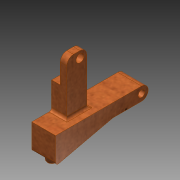
# Autodesk Inventor part: Swinging_connection
Saved by Autodesk Inventor 2015 (Build 190159000, 159)
## iProperties
Created: 2017-02-21
Part Number: Swinging_connection
Material: Wood (Cherry)
Document SubType Name: Modeling
Designer: Guy
Density: 0.63 g/cm^3
Appearance: Cherry - Natural Low Gloss
Author: Guy
Autodesk Inventor part; units mm, degrees
ref_plane "YZ Plane" through (0, 0, 0) normal (1, 0, 0) x (0, 1, 0)
ref_plane "XZ Plane" through (0, 0, 0) normal (0, 1, 0) x (-1, 0, 0)
ref_plane "XY Plane" through (0, 0, 0) normal (0, 0, 1) x (1, 0, 0)
sketch "Sketch1" plane through (0, 0, 0) normal (0, 0, 1) x (1, 0, 0)
  line L0 (0, 0) -> (-70, 0)
  line L1 (0, 0) -> (0, -10)
  line L2 (0, -10) -> (-26.6667, -10)
  line L3 (-26.6667, -10) -> (-70, -20)
  line L4 (-70, -20) -> (-70, 0)
  circle A0 centre (-5, -5) radius 2.5
  dimension "d0" = 70
  dimension "d1" = 5
  dimension "d2" = 10
  dimension "d3" = 5
  dimension "d4" = 5
  dimension "d5" = 20
  constraints: 10 end point, 2 horizontal, 1 centre point, 1 perpendicular, 1 point on line, 1 vertical
  measures "d0" distance of L0.start L0.end
  measures "d1" diameter of A0
  measures "d2" distance between parallel lines of L2 L0
  measures "d3" distance from line of A0.centre L0
  measures "d4" distance from line of A0.centre L1
  measures "d5" distance of L3.end L0.end
extrude "Extrusion1" add sketch "Sketch1" along normal blind 18
fillet "Fillet4" radius 4 1 edges at (-26.6667, -10, 9)
fillet "Fillet5" radius 5 2 edges at (0, 0, 9) (0, -10, 9)
sketch "Sketch4" plane through (-70, -20, 0) normal (0.2248595, -0.9743912, 0) x (0.9743912, 0.2248595, 0)
  circle A0 centre (6, 9) radius 4
  line L0 (44.0167, 18) -> (44.0167, 0) projected
  line L1 (0, 18) -> (44.0167, 18) projected
  line L2 (0, 0) -> (0, 18) projected
  line L3 (0, 0) -> (44.0167, 0) projected
  point P0 (72.7046, 0)
  dimension "d24" = 8
  dimension "d25" = 6
  dimension "d26" = 9
  constraints: 1 centre point
  measures "d24" diameter of A0
  measures "d25" distance from line of L2 A0.centre
  measures "d26" distance from line of L1 A0.centre
extrude "Extrusion4" add sketch "Sketch4" along normal blind 5 contours A0
fillet "Fillet6" radius 1 1 edges at (-66.9269, -24.4222, 9)
sketch "Sketch5" plane through (-70, 0, 0) normal (0, 1, 0) x (1, 0, 0)
  line L0 (15, 0) -> (30, 0)
  line L1 (30, 0) -> (30, -11.5)
  line L2 (30, -11.5) -> (15, -11.5)
  line L3 (15, -11.5) -> (15, 0)
  line L4 (65, -18) -> (0, -18) projected
  line L5 (0, 0) -> (0, -18) projected
  line L6 (65, 0) -> (0, 0) projected
  point P0 (70, 0)
  point P1 (0, -3.5)
  dimension "d31" = 15
  dimension "d33" = 6.5
  dimension "d34" = 15
  constraints: 8 end point, 2 parallel, 1 horizontal, 1 perpendicular, 1 point on line
  measures "d31" distance between parallel lines of L3 L1
  measures "d33" distance between parallel lines of L4 L2
  measures "d34" distance between parallel lines of L5 L3
extrude "Extrusion5" add sketch "Sketch5" along normal blind 40
sketch "Sketch6" plane through (-40, 0, 11.5) normal (0, 0, 1) x (1, 0, 0)
  circle A0 centre (-5, 35) radius 3
  line L0 (-15, 40) -> (0, 40) projected
  line L1 (0, 0) -> (0, 40) projected
  point P0 (40, 0)
  dimension "d37" = 6
  dimension "d38" = 5
  dimension "d39" = 5
  constraints: 1 centre point
  measures "d37" diameter of A0
  measures "d38" distance from line of A0.centre L0
  measures "d39" distance from line of A0.centre L1
extrude "Extrusion6" cut sketch "Sketch6" against normal up to next
sketch "Sketch7" plane through (-55, 0, 0) normal (-1, 0, 0) x (0, 0, 1)
  line L0 (0, 40) -> (6.5, 40)
  line L1 (0, 20) -> (0, 40)
  line L2 (6.5, 40) -> (6.5, 20)
  line L3 (6.5, 20) -> (0, 20)
  line L4 (0, 0) -> (0, 40) projected
  line L5 (11.5, 0) -> (11.5, 40) projected
  line L6 (0, 40) -> (11.5, 40) projected
  dimension "d42" = 5
  dimension "d44" = 20
  constraints: 8 end point, 2 parallel, 1 horizontal, 1 perpendicular, 1 vertical
  measures "d42" distance between parallel lines of L5 L2
  measures "d44" distance from line of L2.end L0
extrude "Extrusion7" cut sketch "Sketch7" against normal up to next
fillet "Fillet8" radius 5 2 edges at (-40, 40, 9) (-55, 40, 9)
fillet "Fillet9" radius 2 3 edges at (-55, 0, 5.75) (-47.5, 0, 11.5) (-40, 0, 5.75)
fillet "Fillet10" radius 2 1 edges at (-70, -20, 9)
body "Solid1"
